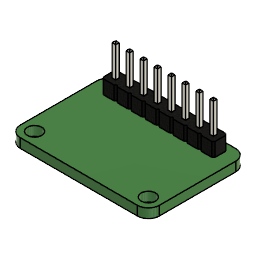
SENSOR DE PRESION v1 (Autodesk Fusion 360 design; units mm, degrees)
Autodesk Fusion 360 part; units mm, degrees
note: some values were not read from the file. Chosen so that the rebuilt part matches the saved one: which bodies a step acts on.
sketch "Boceto1" plane through (0, 0, 0) normal (0, 0, 1) x (1, 0, 0)
  line L0 (2, 0) -> (23.3, 0)
  line L1 (25.3, 2) -> (25.3, 15.9)
  line L2 (23.3, 17.9) -> (2, 17.9)
  line L3 (0, 15.9) -> (0, 2)
  circle A0 centre (23, 2.3) radius 1.3
  arc A1 (23.3, 0) -> (25.3, 2) centre (23.3, 2) ccw
  arc A2 (25.3, 15.9) -> (23.3, 17.9) centre (23.3, 15.9) ccw
  arc A3 (2, 17.9) -> (0, 15.9) centre (2, 15.9) ccw
  arc A4 (0, 2) -> (2, 0) centre (2, 2) ccw
  circle A5 centre (2.3, 2.3) radius 1.3
  line L4 (3.435, 15.275) -> (4.085, 15.275)
  line L5 (4.085, 15.275) -> (4.085, 15.925)
  line L6 (4.085, 15.925) -> (3.435, 15.925)
  line L7 (3.435, 15.925) -> (3.435, 15.275)
  line L8 (3.435, 15.6) -> (4.085, 15.6) construction
  line L9 (5.975, 15.275) -> (6.625, 15.275)
  line L10 (5.975, 15.925) -> (5.975, 15.275)
  line L11 (6.625, 15.925) -> (5.975, 15.925)
  line L12 (6.625, 15.275) -> (6.625, 15.925)
  line L13 (8.515, 15.275) -> (9.165, 15.275)
  line L14 (8.515, 15.925) -> (8.515, 15.275)
  line L15 (9.165, 15.925) -> (8.515, 15.925)
  line L16 (9.165, 15.275) -> (9.165, 15.925)
  line L17 (11.055, 15.275) -> (11.705, 15.275)
  line L18 (11.055, 15.925) -> (11.055, 15.275)
  line L19 (11.705, 15.925) -> (11.055, 15.925)
  line L20 (11.705, 15.275) -> (11.705, 15.925)
  line L21 (13.595, 15.275) -> (14.245, 15.275)
  line L22 (13.595, 15.925) -> (13.595, 15.275)
  line L23 (14.245, 15.925) -> (13.595, 15.925)
  line L24 (14.245, 15.275) -> (14.245, 15.925)
  line L25 (16.135, 15.275) -> (16.785, 15.275)
  line L26 (16.135, 15.925) -> (16.135, 15.275)
  line L27 (16.785, 15.925) -> (16.135, 15.925)
  line L28 (16.785, 15.275) -> (16.785, 15.925)
  line L29 (18.675, 15.275) -> (19.325, 15.275)
  line L30 (18.675, 15.925) -> (18.675, 15.275)
  line L31 (19.325, 15.925) -> (18.675, 15.925)
  line L32 (19.325, 15.275) -> (19.325, 15.925)
  line L33 (21.215, 15.275) -> (21.865, 15.275)
  line L34 (21.215, 15.925) -> (21.215, 15.275)
  line L35 (21.865, 15.925) -> (21.215, 15.925)
  line L36 (21.865, 15.275) -> (21.865, 15.925)
  line L37 (12.65, 17.9) -> (12.65, 0) construction
  point P0 (25.3, 0)
  point P1 (0, 17.9)
  dimension "d1" = 25.3
  dimension "d2" = 17.9
  dimension "d3" = 2.6
  dimension "d4" = 2.3
  dimension "d5" = 2.3
  dimension "d6" = 2
  dimension "d9" = -20.7
  dimension "d10" = 13.3
  dimension "d13" = 0.65
  dimension "d14" = 0.65
  dimension "d15" = 2.3
  dimension "d18" = 17.78
  dimension "d19" = 0
  dimension "d20" = 0.945
  constraint horizontal L0
  constraint vertical L1
  constraint horizontal L2
  constraint vertical L3
  constraint coincident P0 L0
  constraint coincident P0 L1
  constraint tangent L0 A1
  constraint tangent L1 A1
  constraint tangent L1 A2
  constraint tangent L2 A2
  constraint equal A1 A2
  constraint coincident P1 L2
  constraint coincident P1 L3
  constraint tangent L2 A3
  constraint tangent L3 A3
  constraint equal A1 A3
  constraint coincident origin L0
  constraint coincident origin L3
  constraint tangent L0 A4
  constraint tangent L3 A4
  constraint equal A1 A4
  constraint horizontal L4
  constraint vertical L5
  constraint horizontal L6
  constraint vertical L7
  constraint midpoint L7 L8.start
  constraint midpoint L5 L8.end
  constraint midpoint L2 L37.start
  constraint midpoint L0 L37.end
  measures "d1" distance of origin P0
  measures "d2" distance of origin P1
  measures "d3" diameter of A0
  measures "d4" distance of L0 A0.centre
  measures "d5" distance of L1 A0.centre
  measures "d6" radius of A1
  measures "d13" distance of L4.start L4.end
  measures "d14" distance of L4.start L6.end
  measures "d15" distance of L2 L8
  measures "d20" distance of L20 L37
extrude "Extruir1" add sketch "Boceto1" along normal blind 1.7 makes body 1
sketch "Boceto3" plane through (0, 0, 1.7) normal (0, 0, 1) x (-1, 0, 0)
  circle A0 centre (-2.3, -2.3) radius 1.3
  arc A1 (0, -2) -> (-2, 0) centre (-2, -2) ccw
  line L0 (-2, 0) -> (-23.3, 0)
  arc A2 (-23.3, 0) -> (-25.3, -2) centre (-23.3, -2) ccw
  line L1 (-25.3, -2) -> (-25.3, -15.9)
  arc A3 (-25.3, -15.9) -> (-23.3, -17.9) centre (-23.3, -15.9) ccw
  line L2 (-23.3, -17.9) -> (-2, -17.9)
  arc A4 (-2, -17.9) -> (0, -15.9) centre (-2, -15.9) ccw
  line L3 (0, -15.9) -> (0, -2)
  line L4 (-14.245, -15.925) -> (-14.245, -15.275)
  line L5 (-14.245, -15.275) -> (-13.595, -15.275)
  line L6 (-13.595, -15.275) -> (-13.595, -15.925)
  line L7 (-13.595, -15.925) -> (-14.245, -15.925)
  line L8 (-16.785, -15.925) -> (-16.785, -15.275)
  line L9 (-16.785, -15.275) -> (-16.135, -15.275)
  line L10 (-16.135, -15.275) -> (-16.135, -15.925)
  line L11 (-16.135, -15.925) -> (-16.785, -15.925)
  line L12 (-11.705, -15.925) -> (-11.705, -15.275)
  line L13 (-11.705, -15.275) -> (-11.055, -15.275)
  line L14 (-11.055, -15.275) -> (-11.055, -15.925)
  line L15 (-11.055, -15.925) -> (-11.705, -15.925)
  line L16 (-3.435, -15.275) -> (-3.435, -15.925)
  line L17 (-3.435, -15.925) -> (-4.085, -15.925)
  line L18 (-4.085, -15.925) -> (-4.085, -15.275)
  line L19 (-4.085, -15.275) -> (-3.435, -15.275)
  line L20 (-6.625, -15.925) -> (-6.625, -15.275)
  line L21 (-6.625, -15.275) -> (-5.975, -15.275)
  line L22 (-5.975, -15.275) -> (-5.975, -15.925)
  line L23 (-5.975, -15.925) -> (-6.625, -15.925)
  line L24 (-19.325, -15.925) -> (-19.325, -15.275)
  line L25 (-19.325, -15.275) -> (-18.675, -15.275)
  line L26 (-18.675, -15.275) -> (-18.675, -15.925)
  line L27 (-18.675, -15.925) -> (-19.325, -15.925)
  line L28 (-21.865, -15.925) -> (-21.865, -15.275)
  line L29 (-21.865, -15.275) -> (-21.215, -15.275)
  line L30 (-21.215, -15.275) -> (-21.215, -15.925)
  line L31 (-21.215, -15.925) -> (-21.865, -15.925)
  line L32 (-9.165, -15.925) -> (-9.165, -15.275)
  line L33 (-9.165, -15.275) -> (-8.515, -15.275)
  line L34 (-8.515, -15.275) -> (-8.515, -15.925)
  line L35 (-8.515, -15.925) -> (-9.165, -15.925)
  circle A5 centre (-23, -2.3) radius 1.3
  line L36 (-4.73, -14.33) -> (-2.79, -14.33)
  line L37 (-2.49, -14.63) -> (-2.49, -16.57)
  line L38 (-2.79, -16.87) -> (-4.73, -16.87)
  line L39 (-5.03, -16.57) -> (-5.03, -14.63)
  line L40 (-2.49, -16.57) -> (-2.79, -16.87)
  line L41 (-4.73, -16.87) -> (-5.03, -16.57)
  line L42 (-5.03, -14.63) -> (-4.73, -14.33)
  line L43 (-2.79, -14.33) -> (-2.49, -14.63)
  line L44 (-5.33, -14.33) -> (-5.03, -14.63)
  line L45 (-7.27, -14.33) -> (-5.33, -14.33)
  line L46 (-7.57, -14.63) -> (-7.27, -14.33)
  line L47 (-7.57, -16.57) -> (-7.57, -14.63)
  line L48 (-7.27, -16.87) -> (-7.57, -16.57)
  line L49 (-5.33, -16.87) -> (-7.27, -16.87)
  line L50 (-5.03, -16.57) -> (-5.33, -16.87)
  line L51 (-5.03, -14.63) -> (-5.03, -16.57)
  line L52 (-7.87, -14.33) -> (-7.57, -14.63)
  line L53 (-9.81, -14.33) -> (-7.87, -14.33)
  line L54 (-10.11, -14.63) -> (-9.81, -14.33)
  line L55 (-10.11, -16.57) -> (-10.11, -14.63)
  line L56 (-9.81, -16.87) -> (-10.11, -16.57)
  line L57 (-7.87, -16.87) -> (-9.81, -16.87)
  line L58 (-7.57, -16.57) -> (-7.87, -16.87)
  line L59 (-7.57, -14.63) -> (-7.57, -16.57)
  line L60 (-10.41, -14.33) -> (-10.11, -14.63)
  line L61 (-12.35, -14.33) -> (-10.41, -14.33)
  line L62 (-12.65, -14.63) -> (-12.35, -14.33)
  line L63 (-12.65, -16.57) -> (-12.65, -14.63)
  line L64 (-12.35, -16.87) -> (-12.65, -16.57)
  line L65 (-10.41, -16.87) -> (-12.35, -16.87)
  line L66 (-10.11, -16.57) -> (-10.41, -16.87)
  line L67 (-10.11, -14.63) -> (-10.11, -16.57)
  line L68 (-12.95, -14.33) -> (-12.65, -14.63)
  line L69 (-14.89, -14.33) -> (-12.95, -14.33)
  line L70 (-15.19, -14.63) -> (-14.89, -14.33)
  line L71 (-15.19, -16.57) -> (-15.19, -14.63)
  line L72 (-14.89, -16.87) -> (-15.19, -16.57)
  line L73 (-12.95, -16.87) -> (-14.89, -16.87)
  line L74 (-12.65, -16.57) -> (-12.95, -16.87)
  line L75 (-12.65, -14.63) -> (-12.65, -16.57)
  line L76 (-15.49, -14.33) -> (-15.19, -14.63)
  line L77 (-17.43, -14.33) -> (-15.49, -14.33)
  line L78 (-17.73, -14.63) -> (-17.43, -14.33)
  line L79 (-17.73, -16.57) -> (-17.73, -14.63)
  line L80 (-17.43, -16.87) -> (-17.73, -16.57)
  line L81 (-15.49, -16.87) -> (-17.43, -16.87)
  line L82 (-15.19, -16.57) -> (-15.49, -16.87)
  line L83 (-15.19, -14.63) -> (-15.19, -16.57)
  line L84 (-18.03, -14.33) -> (-17.73, -14.63)
  line L85 (-19.97, -14.33) -> (-18.03, -14.33)
  line L86 (-20.27, -14.63) -> (-19.97, -14.33)
  line L87 (-20.27, -16.57) -> (-20.27, -14.63)
  line L88 (-19.97, -16.87) -> (-20.27, -16.57)
  line L89 (-18.03, -16.87) -> (-19.97, -16.87)
  line L90 (-17.73, -16.57) -> (-18.03, -16.87)
  line L91 (-17.73, -14.63) -> (-17.73, -16.57)
  line L92 (-20.57, -14.33) -> (-20.27, -14.63)
  line L93 (-22.51, -14.33) -> (-20.57, -14.33)
  line L94 (-22.81, -14.63) -> (-22.51, -14.33)
  line L95 (-22.81, -16.57) -> (-22.81, -14.63)
  line L96 (-22.51, -16.87) -> (-22.81, -16.57)
  line L97 (-20.57, -16.87) -> (-22.51, -16.87)
  line L98 (-20.27, -16.57) -> (-20.57, -16.87)
  line L99 (-20.27, -14.63) -> (-20.27, -16.57)
  point P0 (-5.03, -14.33)
  point P1 (-2.49, -14.33)
  point P2 (-2.49, -16.87)
  point P3 (-5.03, -16.87)
  dimension "d22" = 0.3
  dimension "d23" = 0.3
  dimension "d24" = 0.3
  dimension "d25" = 0.3
  dimension "d26" = 0.3
  dimension "d27" = 0.3
  dimension "d28" = 0.3
  dimension "d29" = 0.3
  dimension "d32" = -17.78
  dimension "d33" = 0
  constraint coincident P2 L37
  constraint coincident P2 L38
  constraint coincident P3 L38
  constraint coincident P3 L39
  constraint coincident P0 L39
  constraint coincident P0 L36
  constraint coincident P1 L36
  constraint coincident P1 L37
  measures "d22" distance of P2 L37.end
  measures "d23" distance of P2 L38.start
  measures "d24" distance of P3 L38.end
  measures "d25" distance of P3 L39.start
  measures "d26" distance of P0 L39.end
  measures "d27" distance of P0 L36.start
  measures "d28" distance of P1 L36.end
  measures "d29" distance of P1 L37.start
extrude "Extruir2" add sketch "Boceto3" along normal blind 2.5 separate body contours L36 L37 L38 L39 L40 L41 L42 L43 L51 | L39 L44 L45 L46 L47 L48 L49 L50 L51 L59 | L47 L52 L53 L54 L55 L56 L57 L58 L59 L67 | L55 L60 L61 L62 L63 L64 L65 L66 L67 L75 | L63 L68 L69 L70 L71 L72 L73 L74 L75 L83 | L71 L76 L77 L78 L79 L80 L81 L82 L83 L91 | L79 L84 L85 L86 L87 L88 L89 L90 L91 L99 | L87 L92 L93 L94 L95 L96 L97 L98 L99 makes body 2
sketch "Boceto4" plane through (0, 0, 4.2) normal (0, 0, 1) x (-1, 0, 0)
  line L0 (-20.27, -16.57) -> (-19.97, -16.87)
  line L1 (-19.97, -16.87) -> (-18.03, -16.87)
  line L2 (-18.03, -16.87) -> (-17.73, -16.57)
  line L3 (-17.73, -16.57) -> (-17.43, -16.87)
  line L4 (-17.43, -16.87) -> (-15.49, -16.87)
  line L5 (-15.49, -16.87) -> (-15.19, -16.57)
  line L6 (-15.19, -16.57) -> (-14.89, -16.87)
  line L7 (-14.89, -16.87) -> (-12.95, -16.87)
  line L8 (-12.95, -16.87) -> (-12.65, -16.57)
  line L9 (-12.65, -16.57) -> (-12.35, -16.87)
  line L10 (-12.35, -16.87) -> (-10.41, -16.87)
  line L11 (-10.41, -16.87) -> (-10.11, -16.57)
  line L12 (-10.11, -16.57) -> (-9.81, -16.87)
  line L13 (-9.81, -16.87) -> (-7.87, -16.87)
  line L14 (-7.87, -16.87) -> (-7.57, -16.57)
  line L15 (-7.57, -16.57) -> (-7.27, -16.87)
  line L16 (-7.27, -16.87) -> (-5.33, -16.87)
  line L17 (-5.33, -16.87) -> (-5.03, -16.57)
  line L18 (-5.03, -16.57) -> (-4.73, -16.87)
  line L19 (-4.73, -16.87) -> (-2.79, -16.87)
  line L20 (-2.79, -16.87) -> (-2.49, -16.57)
  line L21 (-2.49, -16.57) -> (-2.49, -14.63)
  line L22 (-2.49, -14.63) -> (-2.79, -14.33)
  line L23 (-2.79, -14.33) -> (-4.73, -14.33)
  line L24 (-4.73, -14.33) -> (-5.03, -14.63)
  line L25 (-5.03, -14.63) -> (-5.33, -14.33)
  line L26 (-5.33, -14.33) -> (-7.27, -14.33)
  line L27 (-7.27, -14.33) -> (-7.57, -14.63)
  line L28 (-7.57, -14.63) -> (-7.87, -14.33)
  line L29 (-7.87, -14.33) -> (-9.81, -14.33)
  line L30 (-9.81, -14.33) -> (-10.11, -14.63)
  line L31 (-10.11, -14.63) -> (-10.41, -14.33)
  line L32 (-10.41, -14.33) -> (-12.35, -14.33)
  line L33 (-12.35, -14.33) -> (-12.65, -14.63)
  line L34 (-12.65, -14.63) -> (-12.95, -14.33)
  line L35 (-12.95, -14.33) -> (-14.89, -14.33)
  line L36 (-14.89, -14.33) -> (-15.19, -14.63)
  line L37 (-15.19, -14.63) -> (-15.49, -14.33)
  line L38 (-15.49, -14.33) -> (-17.43, -14.33)
  line L39 (-17.43, -14.33) -> (-17.73, -14.63)
  line L40 (-17.73, -14.63) -> (-18.03, -14.33)
  line L41 (-18.03, -14.33) -> (-19.97, -14.33)
  line L42 (-19.97, -14.33) -> (-20.27, -14.63)
  line L43 (-20.27, -14.63) -> (-20.57, -14.33)
  line L44 (-20.57, -14.33) -> (-22.51, -14.33)
  line L45 (-22.51, -14.33) -> (-22.81, -14.63)
  line L46 (-22.81, -14.63) -> (-22.81, -16.57)
  line L47 (-22.81, -16.57) -> (-22.51, -16.87)
  line L48 (-22.51, -16.87) -> (-20.57, -16.87)
  line L49 (-20.57, -16.87) -> (-20.27, -16.57)
  line L50 (-21.215, -15.275) -> (-21.215, -15.925)
  line L51 (-21.215, -15.925) -> (-21.865, -15.925)
  line L52 (-21.865, -15.925) -> (-21.865, -15.275)
  line L53 (-21.865, -15.275) -> (-21.215, -15.275)
  line L54 (-8.515, -15.275) -> (-8.515, -15.925)
  line L55 (-8.515, -15.925) -> (-9.165, -15.925)
  line L56 (-9.165, -15.925) -> (-9.165, -15.275)
  line L57 (-9.165, -15.275) -> (-8.515, -15.275)
  line L58 (-11.055, -15.275) -> (-11.055, -15.925)
  line L59 (-11.055, -15.925) -> (-11.705, -15.925)
  line L60 (-11.705, -15.925) -> (-11.705, -15.275)
  line L61 (-11.705, -15.275) -> (-11.055, -15.275)
  line L62 (-5.975, -15.275) -> (-5.975, -15.925)
  line L63 (-5.975, -15.925) -> (-6.625, -15.925)
  line L64 (-6.625, -15.925) -> (-6.625, -15.275)
  line L65 (-6.625, -15.275) -> (-5.975, -15.275)
  line L66 (-13.595, -15.275) -> (-13.595, -15.925)
  line L67 (-13.595, -15.925) -> (-14.245, -15.925)
  line L68 (-14.245, -15.925) -> (-14.245, -15.275)
  line L69 (-14.245, -15.275) -> (-13.595, -15.275)
  line L70 (-4.085, -15.925) -> (-4.085, -15.275)
  line L71 (-4.085, -15.275) -> (-3.435, -15.275)
  line L72 (-3.435, -15.275) -> (-3.435, -15.925)
  line L73 (-3.435, -15.925) -> (-4.085, -15.925)
  line L74 (-18.675, -15.275) -> (-18.675, -15.925)
  line L75 (-18.675, -15.925) -> (-19.325, -15.925)
  line L76 (-19.325, -15.925) -> (-19.325, -15.275)
  line L77 (-19.325, -15.275) -> (-18.675, -15.275)
  line L78 (-16.135, -15.275) -> (-16.135, -15.925)
  line L79 (-16.135, -15.925) -> (-16.785, -15.925)
  line L80 (-16.785, -15.925) -> (-16.785, -15.275)
  line L81 (-16.785, -15.275) -> (-16.135, -15.275)
extrude "Extruir3" add sketch "Boceto4" along normal blind 5.75 separate body contours L50 L51 L52 L53 | L54 L55 L56 L57 | L58 L59 L60 L61 | L62 L63 L64 L65 | L66 L67 L68 L69 | L70 L71 L72 L73 | L74 L75 L76 L77 | L78 L79 L80 L81 makes body 3 at (16.135, 15.4917, 6.1167) makes body 4 at (6.4083, 15.275, 6.1167) makes body 5 at (8.515, 15.4917, 6.1167) makes body 6 at (18.8917, 15.925, 6.1167) makes body 7 at (13.595, 15.4917, 6.1167) makes body 8 at (3.8683, 15.275, 6.1167) makes body 9 at (11.055, 15.4917, 6.1167) makes body 10 at (21.215, 15.4917, 6.1167)
extrude "Extruir4" add 1 faces at (3.8683, 15.4917, 4.2) along direction (0, 0, -1) blind 6 on bodies 8 bodies 8
extrude "Extruir5" add 1 faces at (6.4083, 15.4917, 4.2) along direction (0, 0, -1) blind 6 on bodies 4 bodies 4
extrude "Extruir6" add 1 faces at (8.9483, 15.4917, 4.2) along direction (0, 0, -1) blind 6 on bodies 5 bodies 5
extrude "Extruir7" add 1 faces at (11.4883, 15.4917, 4.2) along direction (0, 0, -1) blind 6 on bodies 9 bodies 9
extrude "Extruir8" add 1 faces at (14.0283, 15.4917, 4.2) along direction (0, 0, -1) blind 6 on bodies 7 bodies 7
extrude "Extruir9" add 1 faces at (16.5683, 15.4917, 4.2) along direction (0, 0, -1) blind 6 on bodies 3 bodies 3
extrude "Extruir10" add 1 faces at (19.1083, 15.4917, 4.2) along direction (0, 0, -1) blind 6 on bodies 6 bodies 6
extrude "Extruir11" add 1 faces at (21.6483, 15.4917, 4.2) along direction (0, 0, -1) blind 6 on bodies 10 bodies 10
chamfer "Chaflán1" distance 0.2 angle 45 16 faces at (3.8683, 15.4917, -1.8) (3.8683, 15.4917, 9.95) (11.4883, 15.4917, -1.8) (11.4883, 15.4917, 9.95) (6.4083, 15.4917, -1.8) (6.4083, 15.4917, 9.95) (14.0283, 15.4917, -1.8) (14.0283, 15.4917, 9.95) (16.5683, 15.4917, -1.8) (16.5683, 15.4917, 9.95) (8.9483, 15.4917, -1.8) (8.9483, 15.4917, 9.95) (19.1083, 15.4917, -1.8) (19.1083, 15.4917, 9.95) (21.6483, 15.4917, -1.8) (21.6483, 15.4917, 9.95) on bodies 3 4 5 6 7 8 9 10
equation "d9 = -25.3 mm + 2.3 mm + 2.3 mm"
equation "d10 = 17.90 mm - 2.3 mm - 2.3 mm"
equation "d18 = ( 2.54 * 7 ) * 1 mm"
equation "d20 = ( 1.89 / 2 ) * 1 mm"
equation "d23 = d22"
equation "d25 = d24"
equation "d27 = d26"
equation "d29 = d28"
equation "d32 = -2.54 * 7 mm"
equation "d38 = 11.25 mm - 5.25 mm"
